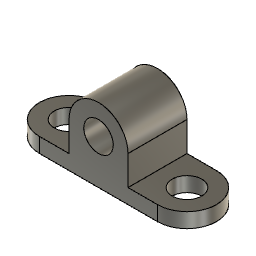
A4 (Autodesk Fusion 360 design; units mm, degrees)
Autodesk Fusion 360 part; units mm, degrees
sketch "Base" plane through (0, 0, 0) normal (0, 0, 1) x (1, 0, 0)
  line L0 (0, 0) -> (80, 0)
  line L1 (0, 0) -> (0, 40)
  line L2 (0, 40) -> (80, 40)
  line L3 (80, 40) -> (80, 0)
  line L4 (0, 0) -> (-20, 0)
  line L5 (-20, 0) -> (-20, 40)
  line L6 (-20, 40) -> (0, 40)
  line L7 (80, 40) -> (100, 40)
  line L8 (100, 40) -> (100, 0)
  line L9 (100, 0) -> (80, 0)
  dimension "d1" = 80
  constraint coincident L0.start L1.start
  constraint horizontal L0
  constraint perpendicular L0 L1
  constraint perpendicular L1 L2
  constraint perpendicular L0 L3
  constraint perpendicular L1 L4
  constraint perpendicular L0 L5
  constraint perpendicular L1 L6
  constraint perpendicular L3 L7
  constraint perpendicular L7 L8
  constraint perpendicular L3 L9
  measures "d1" distance of L0.start L0.end
extrude "Extrude1" add sketch "Base" along normal blind 10
fillet "Fillet1" radius 20 4 edges at (100, 40, 5) (100, 0, 5) (-20, 0, 5) (-20, 40, 5)
sketch "side holes" plane through (0, 0, 10) normal (0, 0, 1) x (-1, 0, 0)
  arc A0 (0, -40) -> (0, 0) centre (0, -20) ccw
  line L0 (0, 0) -> (-80, 0)
  arc A1 (-80, 0) -> (-80, -40) centre (-80, -20) ccw
  line L1 (-80, -40) -> (0, -40)
  circle A2 centre (0, -20) radius 10
  line L2 (20, -20) -> (10, -20)
  line L3 (-40, -40) -> (-40, 5)
  circle A3 centre (-80, -20) radius 10
  constraint midpoint A0 L2.start
  constraint horizontal L2
  constraint coincident A0.centre A2.centre
  constraint midpoint L1 L3.start
  constraint perpendicular L0 L3
  constraint symmetric A2 L3 A3
extrude "Extrude2" cut sketch "side holes" against normal blind 10 contours A2 | A3
sketch "inner base" plane through (0, 0, 10) normal (0, 0, 1) x (-1, 0, 0)
  circle A0 centre (0, -20) radius 10
  circle A1 centre (-80, -20) radius 10
  arc A2 (0, -40) -> (0, 0) centre (0, -20) ccw
  line L0 (0, 0) -> (-80, 0)
  arc A3 (-80, 0) -> (-80, -40) centre (-80, -20) ccw
  line L1 (-80, -40) -> (0, -40)
  line L2 (0, 0) -> (-20, 0)
  line L3 (-20, 0) -> (-60, 0)
  line L4 (-20, 0) -> (-20, -40)
  line L5 (-60, -40) -> (-60, 0)
  constraint coincident A2.end L0.start
  constraint coincident L0 L2.end
  constraint coincident L0 L3.end
  constraint coincident L1 L4.end
  constraint perpendicular L1 L4
  constraint coincident L1 L5.start
  constraint perpendicular L3 L5
extrude "Extrude3" add sketch "inner base" along normal blind 40 contours L0 L1 L3 L4 L5
fillet "Fillet2" radius 20 2 edges at (20, 20, 50) (60, 20, 50)
sketch "middle hole" plane through (0, 0, 0) normal (0, -1, 0) x (1, 0, 0)
  arc A0 (60, 30) -> (20, 30) centre (40, 30) ccw
  line L0 (20, 30) -> (20, 10)
  line L1 (20, 10) -> (0, 10)
  line L2 (0, 10) -> (0, 0)
  line L3 (0, 0) -> (80, 0)
  line L4 (80, 0) -> (80, 10)
  line L5 (80, 10) -> (60, 10)
  line L6 (60, 10) -> (60, 30)
  circle A1 centre (40, 30) radius 10
  line L7 (40, 50) -> (40, 40)
  constraint concentric A0 A1
  constraint midpoint A0 L7.start
  constraint vertical L7
extrude "Extrude4" cut sketch "middle hole" against normal blind 40 contours A1
named bodies: "main body"
